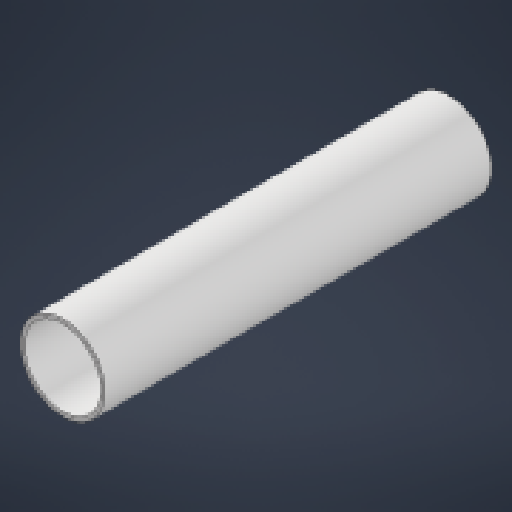
# Autodesk Inventor part: 导管
Saved by Autodesk Inventor 2025 (Build 290162000, 162)
## iProperties
Created: 2024-05-12
Part Number: 导管
Material: 常规
Document SubType Name: Modeling
Designer: HZD
Density: 1 g/cm^3
Appearance: 默认
Author: HZD
Autodesk Inventor part; units mm, degrees
ref_plane "YZ Plane" through (0, 0, 0) normal (1, 0, 0) x (0, 1, 0)
ref_plane "XZ Plane" through (0, 0, 0) normal (0, 1, 0) x (-1, 0, 0)
ref_plane "XY Plane" through (0, 0, 0) normal (0, 0, 1) x (1, 0, 0)
sketch "草图1" plane through (0, 0, 0) normal (0, 0, 1) x (1, 0, 0)
  circle A0 centre (0, 0) radius 10
  circle A1 centre (0, 0) radius 9
  dimension "d0" = 20
  dimension "d1" = 1
  dimension "d4" = 18
  constraints: 2 centre point, 1 coincident
  measures "d0" diameter of A0
  measures "d1" radial gap between concentric circles of A0 A1
  measures "d4" diameter of A1
extrude "拉伸1" add sketch "草图1" along normal blind 91
